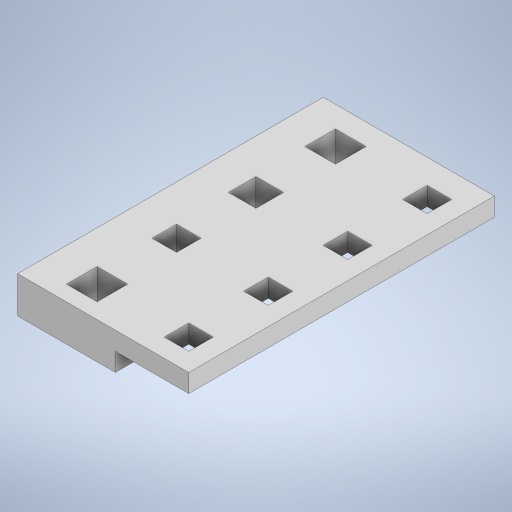
# Autodesk Inventor part: Part14
Saved by Autodesk Inventor 2023 (Build 270158000, 158)
## iProperties
Created: 2024-12-09
Part Number: Part14
Material: Generic
Document SubType Name: Sheet Metal
Designer: 1ZHUSAM
Density: 1 g/cm^3
Sheet Metal Rule: Default_mm
Appearance: Default
Author: 1ZHUSAM
Autodesk Inventor part; units mm, degrees
ref_plane "YZ Plane" through (0, 0, 0) normal (1, 0, 0) x (0, 1, 0)
ref_plane "XZ Plane" through (0, 0, 0) normal (0, 1, 0) x (-1, 0, 0)
ref_plane "XY Plane" through (0, 0, 0) normal (0, 0, 1) x (1, 0, 0)
sketch "Sketch1" plane through (0, 0, 0) normal (0, 1, 0) x (-1, 0, 0)
  line L0 (0, 0) -> (0, -50)
  line L1 (0, -50) -> (-10, -50)
  line L2 (-10, -50) -> (-10, 0)
  line L3 (-10, 0) -> (0, 0)
  line L4 (-5, -50) -> (-5, -46)
  line L5 (-5, -46) -> (-3, -46)
  line L6 (-3, -46) -> (-3, -42)
  line L7 (-3, -42) -> (-7, -42)
  line L8 (-7, -42) -> (-7, -46)
  line L9 (-7, -46) -> (-5, -46)
  line L10 (-5, -42) -> (-5, -33)
  line L11 (-5, -33) -> (-7, -33)
  line L12 (-7, -33) -> (-7, -29)
  line L13 (-7, -29) -> (-3, -29)
  line L14 (-3, -29) -> (-3, -33)
  line L15 (-5, -33) -> (-3, -33)
  line L16 (-5, -29) -> (-5, -20)
  line L17 (-5, -20) -> (-3, -20)
  line L18 (-3, -20) -> (-3, -16)
  line L19 (-3, -16) -> (-7, -16)
  line L20 (-7, -16) -> (-7, -20)
  line L21 (-5, -20) -> (-7, -20)
  line L22 (-5, -16) -> (-5, -7)
  line L23 (-5, -7) -> (-7, -7)
  line L24 (-7, -7) -> (-7, -3)
  line L25 (-7, -3) -> (-3, -3)
  line L26 (-5, -7) -> (-3, -7)
  line L27 (-3, -7) -> (-3, -3)
  line L28 (0, -50) -> (2, -50)
  line L29 (2, -50) -> (2, 0)
  line L30 (2, 0) -> (0, 0)
  dimension "d0" = 50
  dimension "d1" = 10
  dimension "d2" = 90
  dimension "d3" = 4
  dimension "d4" = 2
  dimension "d5" = 4
  dimension "d6" = 4
  dimension "d7" = 9
  dimension "d8" = 4
  dimension "d9" = 9
  dimension "d10" = 4
  dimension "d11" = 9
  dimension "d12" = 4
  dimension "d13" = 2
  constraints: 62 end point, 17 point on line, 16 perpendicular, 4 midpoint, 3 horizontal, 3 vertical
  measures "d0" distance of L0.start L0.end
  measures "d1" distance of L0.end L1.end
  measures "d2" angle of L1 L2
  measures "d3" distance of L4.start L4.end
  measures "d4" distance of L4.end L5.end
  measures "d5" distance of L5.end L6.end
  measures "d6" distance of L6.end L7.end
  measures "d7" distance of L10.start L10.end
  measures "d8" distance of L11.end L12.end
  measures "d9" distance of L16.start L16.end
  measures "d10" distance of L17.end L18.end
  measures "d11" distance of L22.start L22.end
  measures "d12" distance of L23.end L24.end
  measures "d13" distance of L0.end L28.end
extrude "Extrusion1" add sketch "Sketch1" along normal blind 3
sketch "Sketch2" plane through (-2, 0, -50) normal (-1, 0, 0) x (0, 0, 1)
  line L0 (0, 0) -> (0, 3) projected
  line L1 (0, 3) -> (50, 3)
  line L2 (50, 3) -> (50, -3)
  line L3 (50, -3) -> (0, -3)
  line L4 (0, -3) -> (0, 3)
  point P0 (50, 0)
  dimension "d16" = 6
  constraints: 8 end point, 2 parallel, 1 horizontal, 1 perpendicular
  measures "d16" distance of L1.end L2.end
extrude "Extrusion2" add sketch "Sketch2" along normal blind 16
sketch "Sketch3" plane through (0, 3, 0) normal (0, 1, 0) x (1, 0, 0)
  line L0 (-2, 0) -> (-18, 0) projected
  line L1 (-10, 0) -> (-10, 50)
  line L2 (10, 50) -> (-18, 50) projected
  line L3 (-12.5, 41.5) -> (-7.5, 41.5)
  line L4 (-7.5, 41.5) -> (-7.5, 46.5)
  line L5 (-7.5, 46.5) -> (-12.5, 46.5)
  line L6 (-12.5, 46.5) -> (-12.5, 41.5)
  line L7 (-12.5, 41.5) -> (-7.5, 46.5) construction
  line L8 (-7.5, 41.5) -> (-12.5, 46.5) construction
  line L9 (-12.5, 2.5) -> (-7.5, 2.5)
  line L10 (-7.5, 2.5) -> (-7.5, 7.5)
  line L11 (-7.5, 7.5) -> (-12.5, 7.5)
  line L12 (-12.5, 7.5) -> (-12.5, 2.5)
  line L13 (-12.5, 2.5) -> (-7.5, 7.5) construction
  line L14 (-7.5, 2.5) -> (-12.5, 7.5) construction
  line L15 (-12, 16) -> (-8, 16)
  line L16 (-8, 16) -> (-8, 20)
  line L17 (-8, 20) -> (-12, 20)
  line L18 (-12, 20) -> (-12, 16)
  line L19 (-12, 16) -> (-8, 20) construction
  line L20 (-8, 16) -> (-12, 20) construction
  line L21 (-12.25, 28.75) -> (-7.75, 28.75)
  line L22 (-7.75, 28.75) -> (-7.75, 33.25)
  line L23 (-7.75, 33.25) -> (-12.25, 33.25)
  line L24 (-12.25, 33.25) -> (-12.25, 28.75)
  line L25 (-12.25, 28.75) -> (-7.75, 33.25) construction
  line L26 (-7.75, 28.75) -> (-12.25, 33.25) construction
  point P0 (0, 0)
  point P1 (-10, 44)
  point P2 (-10, 5)
  point P3 (-10, 18)
  point P4 (-10, 31)
  dimension "d19" = 5
  dimension "d20" = 5
  dimension "d21" = 5
  dimension "d22" = 5
  dimension "d23" = 4
  dimension "d24" = 4
  dimension "d25" = 4.5
  dimension "d26" = 4.5
  constraints: 50 end point, 9 midpoint, 8 parallel, 5 point on line, 4 horizontal, 4 perpendicular, 1 vertical
  measures "d19" distance of L5.end L4.end
  measures "d20" distance of L4.end L3.end
  measures "d21" distance of L11.end L10.end
  measures "d22" distance of L10.end L9.end
  measures "d23" distance of L17.end L16.end
  measures "d24" distance of L16.end L15.end
  measures "d25" distance of L23.end L22.end
  measures "d26" distance of L22.end L21.end
extrude "Extrusion3" cut sketch "Sketch3" against normal blind 16
sketch "Sketch4" plane through (-2, -3, -50) normal (0, -1, 0) x (1, 0, 0)
  point P0 (2, 50)
equation "\"BendRadius\" = Thickness"
equation "\"BendReliefWidth\" = Thickness"
equation "\"BendReliefDepth\" = 0.5 * Thickness"
equation "\"CornerReliefSize\" = 4 * Thickness"
equation "\"MinimumRemnant\" = 2 * Thickness"
equation "\"TransitionRadius\" = BendRadius"
equation "\"JacobiRadiusSize\" = BendRadius"
equation "\"GapSize\" = Thickness"
equation "\"Thickness\" = 0.5"
body "Solid1"
